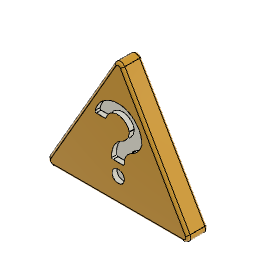
CautionSign (Autodesk Fusion 360 design; units mm, degrees)
Autodesk Fusion 360 part; units mm, degrees
note: some values were not read from the file. Set by a fixed rule: which sketch regions a step uses.
sketch "Sketch1" plane through (0, 0, 0) normal (0, 1, 0) x (1, 0, 0)
  line L0 (2.1997, -3.81) -> (35.9003, -62.1811)
  line L1 (4.3994, 0) -> (71.8006, 0) construction
  line L2 (40.2997, -62.1811) -> (74.0003, -3.81)
  line L3 (76.2, 0) -> (0, 0)
  arc A0 (35.9003, -62.1811) -> (40.2997, -62.1811) centre (38.1, -60.9111) ccw
  arc A1 (74.0003, -3.81) -> (71.8006, 0) centre (71.8006, -2.54) ccw
  arc A2 (4.3994, 0) -> (2.1997, -3.81) centre (4.3994, -2.54) ccw
  point P0 (38.1, -65.9911)
  point P1 (76.2, 0)
  dimension "d1" = 60
  dimension "d2" = 76.2
  dimension "d4" = 76.2
  dimension "d7" = 2.54
  dimension "d8" = 2.54
  constraint horizontal L1
  constraint coincident L3.end origin
  constraint coincident P0 L0
  constraint coincident P0 L2
  constraint tangent L0 A0
  constraint tangent L2 A0
  constraint coincident P1 L1
  constraint coincident P1 L2
  constraint tangent L1 A1
  constraint tangent L2 A1
  constraint coincident L3.end L0
  constraint coincident L3.end L1
  constraint tangent L0 A2
  constraint tangent L1 A2
  constraint equal A1 A2
  measures "d1" angle of L0 L1
  measures "d2" distance of L3.end P0
  measures "d4" distance of P0 P1
  measures "d7" radius of A0
  measures "d8" radius of A1
extrude "Extrude1" add sketch "Sketch1" along normal blind 12.7
sketch "Sketch2" plane through (0, 0, 0) normal (0, -1, 0) x (1, 0, 0)
  arc A0 (2.1997, 3.81) -> (4.3994, 0) centre (4.3994, 2.54) ccw
  line L0 (4.3994, 0) -> (71.8006, 0)
  arc A1 (71.8006, 0) -> (74.0003, 3.81) centre (71.8006, 2.54) ccw
  line L1 (74.0003, 3.81) -> (40.2997, 62.1811)
  arc A2 (40.2997, 62.1811) -> (35.9003, 62.1811) centre (38.1, 60.9111) ccw
  line L2 (35.9003, 62.1811) -> (2.1997, 3.81)
  circle A3 centre (38.1, 12.7) radius 3.175
  line L3 (31.2844, 35.295) -> (26.7797, 35.295)
  arc A4 (43.8189, 35.3736) -> (31.8923, 35.7466) centre (37.8056, 33.9623) ccw
  arc A5 (50.3635, 32.7617) -> (26.1659, 36.0926) centre (38.0602, 32.9416) ccw
  arc A6 (39.4129, 29.0927) -> (43.8356, 35.2148) centre (37.1886, 35.3581) ccw
  arc A7 (45.1318, 26.343) -> (50.3389, 32.5958) centre (40.6355, 35.382) ccw
  arc A8 (39.4129, 29.0927) -> (34.8601, 19.4443) centre (44.4732, 20.8065) ccw
  arc A9 (45.1318, 26.343) -> (41.228, 19.5734) centre (48.2777, 20.0185) ccw
  line L4 (35.4888, 18.8984) -> (40.5943, 18.8984)
  arc A10 (26.1659, 36.0926) -> (26.7797, 35.295) centre (26.7797, 35.93) ccw
  arc A11 (31.2844, 35.295) -> (31.8923, 35.7466) centre (31.2844, 35.93) ccw
  arc A12 (34.8601, 19.4443) -> (35.4888, 18.8984) centre (35.4888, 19.5334) ccw
  arc A13 (40.5943, 18.8984) -> (41.228, 19.5734) centre (40.5943, 19.5334) ccw
  arc A14 (43.8356, 35.2148) -> (43.8189, 35.3736) centre (43.2007, 35.2285) ccw
  arc A15 (50.3389, 32.5958) -> (50.3635, 32.7617) centre (49.7286, 32.771) ccw
  point P0 (34.9534, 18.8984)
  point P1 (41.3034, 18.8984)
  dimension "d9" = 6.35
  dimension "d11" = 6.35
  dimension "d12" = 0.635
  constraint tangent A6 A7
  constraint tangent A7 A9
  constraint horizontal L4
  constraint tangent L3 A10
  constraint tangent A5 A10
  constraint tangent L3 A11
  constraint tangent A4 A11
  constraint equal A10 A11
  constraint coincident P0 L4
  constraint coincident P0 A8
  constraint tangent A8 A12
  constraint tangent L4 A12
  constraint equal A10 A12
  constraint coincident P1 L4
  constraint coincident A9 P1
  constraint tangent L4 A13
  constraint tangent A9 A13
  constraint equal A10 A13
  constraint tangent A4 A14
  constraint tangent A6 A14
  constraint equal A10 A14
  constraint tangent A5 A15
  constraint tangent A7 A15
  constraint equal A10 A15
  measures "d9" diameter of A3
  measures "d11" distance of P0 P1
  measures "d12" radius of A10
extrude "Extrude2" cut 1 faces at (38.8332, 12.7, 20.727) along direction (0, -1, 0) blind 2.54
extrude "Extrude3" cut sketch "Sketch2" against normal blind 2.54 contours A3 | L3 A4 A5 A6 A7 A8 A9 L4 A10 A11 A12 A13 A14 A15
fillet "Fillet1" radius 1.27 6 edges at (38.1, 0, 0) (2.1997, 0, 1.27) (19.05, 0, 32.9956) (38.1, 0, 63.4511) (57.15, 0, 32.9956) (74.0003, 0, 1.27)
fillet "Fillet2" radius 1.27 6 edges at (19.05, 10.16, 32.9956) (2.1997, 10.16, 1.27) (38.1, 10.16, 0) (74.0003, 10.16, 1.27) (57.15, 10.16, 32.9956) (38.1, 10.16, 63.4511)
